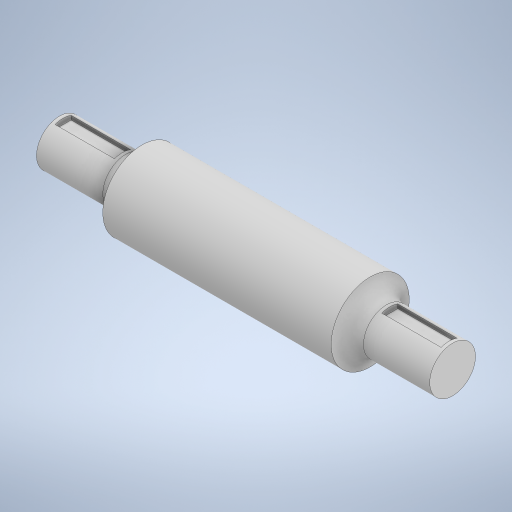
# Autodesk Inventor part: EJE_CUÑEROS
Saved by Autodesk Inventor 2024 (Build 280153000, 153)
## iProperties
Created: 2024-03-01
Part Number: EJE_CUÑEROS
Material: Generic
Document SubType Name: Modeling
Designer: augus
Mass: 106.669 g
Surface Area: 149.312 cm^2
Volume: 106.669 cm^3
Density: 1 g/cm^3
Appearance: Default
Author: augus
Autodesk Inventor part; units mm, degrees
ref_plane "YZ Plane" through (0, 0, 0) normal (1, 0, 0) x (0, 1, 0)
ref_plane "XY Plane" through (0, 0, 0) normal (0, 0, 1) x (1, 0, 0)
sketch "Sketch1" plane through (0, 0, 0) normal (0, 0, 1) x (1, 0, 0)
  line L0 (-7.0711, 17.0711) -> (-57.0711, 17.0711)
  arc A0 (-7.0711, 17.0711) -> (0, 10) centre (0, 17.0711) ccw
  line L1 (0, 10) -> (14.502, 10)
  line L2 (14.502, 0) -> (0, 0)
  arc A1 (-114.1421, 10) -> (-107.0711, 17.0711) centre (-114.1421, 17.0711) ccw
  line L3 (-114.1421, 10) -> (-128.6441, 10)
  line L4 (-128.6441, 0) -> (-114.1421, 0)
  line L5 (-114.1421, 0) -> (0, 0)
  line L6 (-107.0711, 17.0711) -> (-57.0711, 17.0711)
  line L7 (-143.1461, 10) -> (-128.6441, 10)
  line L8 (-128.6441, 0) -> (-143.1461, 0)
  line L9 (-143.1461, 10) -> (-143.1461, 0)
  line L10 (29.0039, 10) -> (14.502, 10)
  line L11 (14.502, 0) -> (29.0039, 0)
  line L12 (29.0039, 10) -> (29.0039, 0)
  constraints: 26 end point, 4 point on circle, 3 horizontal, 2 centre point, 2 parallel, 2 vertical
revolve "Revolution1" add sketch "Sketch1" angle 360 about axis through (-114.1421, 0, 0) along (1, 0, 0)
ref_plane "Work Plane1" through (14.502, 10, 0) normal (0, 1, 0) x (-1, 0, 0)
sketch "Sketch3" plane through (14.502, 10, 0) normal (0, 1, 0) x (-1, 0, 0)
  line L0 (14.502, 0) -> (-14.502, 0)
  line L1 (-14.502, 10) -> (-14.502, -10) projected
  line L2 (13, -3.5) -> (-13, -3.5)
  line L3 (-13, -3.5) -> (-13, 3.5)
  line L4 (-13, 3.5) -> (13, 3.5)
  line L5 (13, 3.5) -> (13, -3.5)
  line L6 (13, -3.5) -> (-13, 3.5) construction
  line L7 (-13, -3.5) -> (13, 3.5) construction
  line L8 (156.0151, -3.5) -> (130.0151, -3.5)
  line L9 (130.0151, -3.5) -> (130.0151, 3.5)
  line L10 (130.0151, 3.5) -> (156.0151, 3.5)
  line L11 (156.0151, 3.5) -> (156.0151, -3.5)
  point P0 (0, 0)
  dimension "d8" = 26
  dimension "d9" = 7
  dimension "d10" = 26
  dimension "d11" = 7
  constraints: 22 end point, 4 midpoint, 4 parallel, 2 horizontal, 2 perpendicular
  measures "d8" distance of L3.end L4.end
  measures "d9" distance of L2.end L3.end
  measures "d10" distance of L10.start L10.end
  measures "d11" distance of L8.end L10.start
extrude "Extrusion1" cut sketch "Sketch3" against normal blind 2.4
body "Solid1"
